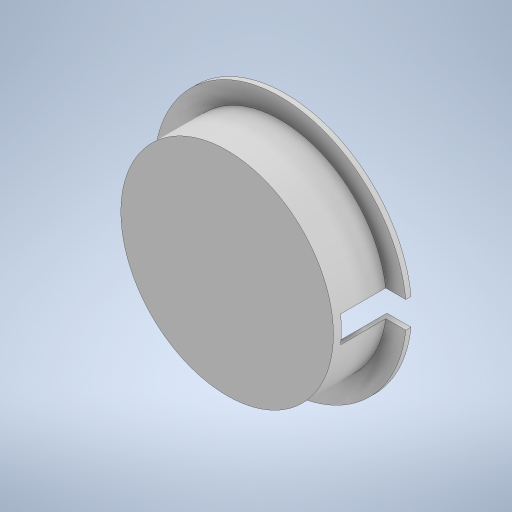
# Autodesk Inventor part: 라이다소켓
Saved by Autodesk Inventor 2024 (Build 280153000, 153)
## iProperties
Created: 2023-09-04
Part Number: 라이다소켓
Material: 일반
Document SubType Name: Modeling
Designer: window
Density: 1 g/cm^3
Appearance: 기본값
Author: window
Autodesk Inventor part; units mm, degrees
ref_plane "YZ Plane" through (0, 0, 0) normal (1, 0, 0) x (0, 1, 0)
ref_plane "XZ Plane" through (0, 0, 0) normal (0, 1, 0) x (-1, 0, 0)
ref_plane "XY Plane" through (0, 0, 0) normal (0, 0, 1) x (1, 0, 0)
sketch "스케치1" plane through (0, 0, 0) normal (0, 0, 1) x (1, 0, 0)
  circle A0 centre (0, 0) radius 38.5
  circle A1 centre (0, 0) radius 40
  dimension "d0" = 77
  dimension "d1" = 80
  constraints: 2 centre point, 2 coincident
  measures "d0" diameter of A0
  measures "d1" diameter of A1
extrude "돌출1" add sketch "스케치1" along normal blind 20 contours A0 | A1
sketch "스케치2" plane through (0, 0, 0) normal (0, 0, -1) x (-1, 0, 0)
  circle A0 centre (0, 0) radius 38.5
  circle A1 centre (0, 0) radius 38.5
  dimension "d4" = 77
  dimension "d7" = 77
  constraints: 2 centre point, 2 coincident
  measures "d4" diameter of A0
  measures "d7" diameter of A1
extrude "돌출2" cut sketch "스케치2" against normal blind 17
sketch "스케치3" plane through (0, 0, 0) normal (0, 0, 1) x (1, 0, 0)
  circle A0 centre (0, 0) radius 38.5
  circle A1 centre (0, 0) radius 47.5
  dimension "d8" = 95
  dimension "d9" = 77
  constraints: 2 centre point, 2 coincident
  measures "d8" diameter of A1
  measures "d9" diameter of A0
extrude "돌출3" add sketch "스케치3" against normal blind 2
sketch "스케치4" plane through (0, 0, -2) normal (0, 0, -1) x (-1, 0, 0)
  line L0 (-25.3897, 5) -> (-51.6103, 5)
  line L1 (-51.6103, 5) -> (-51.6103, -5)
  line L2 (-51.6103, -5) -> (-25.3897, -5)
  line L3 (-25.3897, -5) -> (-25.3897, 5)
  circle A0 centre (0, 0) radius 38.5 projected
  line L4 (-25.3897, 5) -> (-51.6103, -5) construction
  line L5 (-51.6103, 5) -> (-25.3897, -5) construction
  point P0 (-38.5, 0)
  dimension "d12" = 26.2206
  dimension "d13" = 10
  constraints: 12 end point, 2 midpoint, 2 parallel, 1 horizontal, 1 horizontal alignment, 1 perpendicular, 1 other
  measures "d12" distance of L1.end L2.end
  measures "d13" distance of L0.end L1.end
extrude "돌출4" cut sketch "스케치4" against normal blind 19 contours L3 L2 A0 L0 | A0 L2 L1 L0 picked at (-29.7477, -0.557)
